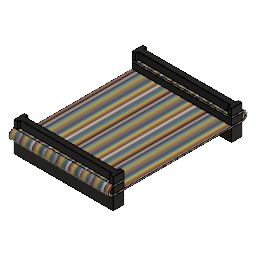
b6c1d7c7-71d5-4f8c-a852-1080e0dc13f3 (Autodesk Fusion 360 design; units mm, degrees)
Autodesk Fusion 360 part; units mm, degrees
note: some values were not read from the file. Set by a fixed rule: which face or edge a step refers to.
sketch "Sketch1" plane through (0, 0, 0) normal (0, 0, 1) x (1, 0, 0) in component "GPIO Header cable v2"
  line L0 (27.75, 3) -> (-27.75, 3)
  line L1 (-27.75, 3) -> (-27.75, -3)
  line L2 (-27.75, -3) -> (27.75, -3)
  line L3 (27.75, -3) -> (27.75, 3)
  line L4 (27.75, 3) -> (-27.75, -3) construction
  line L5 (-27.75, 3) -> (27.75, -3) construction
  line L6 (-1.925, -3) -> (1.925, -3)
  line L7 (1.925, -3) -> (1.925, -3.8)
  line L8 (1.925, -3.8) -> (-1.925, -3.8)
  line L9 (-1.925, -3.8) -> (-1.925, -3)
  dimension "d1" = 55.5
  dimension "d2" = 6
  dimension "d3" = 3.85
  dimension "d4" = 0.8
  constraint perpendicular L0 L1
  constraint parallel L0 L2
  constraint parallel L1 L3
  constraint horizontal L0
  constraint coincident L4 origin
  constraint coincident L5 origin
  constraint horizontal L6
  constraint vertical L7
  constraint horizontal L8
  constraint vertical L9
  constraint midpoint L2 L6
  measures "d1" distance of L1.end L2.end
  measures "d2" distance of L0.end L1.end
  measures "d3" distance of L6.start L6.end
  measures "d4" distance of L6.start L8.end
extrude "Extrude1" add sketch "Sketch1" along normal blind 7 makes body 1 in component "GPIO Header cable v2"
sketch "Sketch2" plane through (0, 0, 7) normal (0, 0, 1) x (-1, 0, 0) in component "GPIO Header cable v2"
  line L0 (-1.925, 3) -> (-27.75, 3)
  line L1 (-27.75, 3) -> (-27.75, -3)
  line L2 (-27.75, -3) -> (27.75, -3)
  line L3 (27.75, -3) -> (27.75, 3)
  line L4 (27.75, 3) -> (1.925, 3)
  line L5 (1.925, 3) -> (1.925, 3.8)
  line L6 (1.925, 3.8) -> (-1.925, 3.8)
  line L7 (-1.925, 3.8) -> (-1.925, 3)
  line L8 (27.75, -3) -> (-27.75, -3)
  line L9 (-27.75, -3) -> (-27.75, 3)
  line L10 (-27.75, 3) -> (27.75, 3)
  line L11 (27.75, 3) -> (27.75, -3)
  constraint horizontal L8
  constraint vertical L9
  constraint horizontal L10
  constraint vertical L11
  constraint coincident L0.end L1.start
  constraint coincident L2.end L3.start
extrude "Extrude2" add sketch "Sketch2" along normal blind 1 separate body contours L0 L1 L2 L3 L4 L8 L9 L10 L11 makes body 2 in component "GPIO Header cable v2"
extrude "Extrude3" add 1 faces at (0.6417, 1, 8) along direction (0, 0, 1) blind 3.5 separate body on bodies 2 makes body 3 in component "GPIO Header cable v2"
extrude "Extrude4" add 1 faces at (0.6417, 1, 11.5) along direction (0, 0, 1) blind 1 separate body on bodies 3 makes body 4 in component "GPIO Header cable v2"
extrude "Extrude5" add 1 faces at (0.6417, 1, 12.5) along direction (0, 0, 1) blind 4 separate body on bodies 4 makes body 5 in component "GPIO Header cable v2"
sketch "Sketch4" plane through (0, 0, 16.5) normal (0, 0, 1) x (-1, 0, 0) in component "GPIO Header cable v2"
  line L0 (27.75, 3) -> (-27.75, 3)
  line L1 (-27.75, 3) -> (-27.75, -3)
  line L2 (-27.75, -3) -> (27.75, -3)
  line L3 (27.75, -3) -> (27.75, 3)
  line L4 (25.625, -3) -> (-25.625, -3)
  line L5 (-25.625, -3) -> (-25.625, -1.5)
  line L6 (-25.625, -1.5) -> (25.625, -1.5)
  line L7 (25.625, -1.5) -> (25.625, -3)
  line L8 (25.625, 1.5) -> (-25.625, 1.5)
  line L9 (-25.625, 1.5) -> (-25.625, 3)
  line L10 (-25.625, 3) -> (25.625, 3)
  line L11 (25.625, 3) -> (25.625, 1.5)
  dimension "d15" = 51.25
  dimension "d16" = 1.5
  dimension "d17" = 1.5
  dimension "d18" = 51.25
  constraint horizontal L4
  constraint vertical L5
  constraint horizontal L6
  constraint vertical L7
  constraint midpoint L2 L4
  constraint horizontal L8
  constraint vertical L9
  constraint horizontal L10
  constraint vertical L11
  constraint midpoint L0 L10
  measures "d15" distance of L4.start L4.end
  measures "d16" distance of L4.start L6.end
  measures "d17" distance of L8.start L10.end
  measures "d18" distance of L8.start L8.end
extrude "Extrude6" cut sketch "Sketch4" against normal blind 4 contours L0 L8 L9 L10 L11 | L2 L4 L5 L6 L7 bodies 5 in component "GPIO Header cable v2"
extrude "Extrude7" add 3 faces at (0.6417, -3, 7.3333) (-19.1417, -3, 7.3333) (10.5333, -3, 7.3333) along direction (0, -1, 0) blind 15 on bodies 2 bodies 2 in component "GPIO Header cable v2"
sketch "Sketch5" plane through (27.75, 0, 0) normal (1, 0, 0) x (0, 1, 0) in component "GPIO Header cable v2"
  line L0 (-3, 8) -> (3, 8)
  line L1 (3, 8) -> (3, 11.5)
  line L2 (3, 11.5) -> (-3, 11.5)
  line L3 (-3, 11.5) -> (-3, 8)
  arc A0 (3, 8) -> (3, 11.5) centre (3, 9.75) ccw
  arc A1 (3, 7) -> (3, 12.5) centre (3, 9.75) ccw
  line L4 (3, 12.5) -> (3, 11.5)
  line L5 (3, 8) -> (3, 7)
  dimension "d23" = 1
  constraint coincident L0.end L1.start
  constraint coincident L1.end L2.start
  constraint tangent L2 A0
  constraint perpendicular L2 L4
  constraint perpendicular L0 L5
extrude "Extrude8" add sketch "Sketch5" against normal blind 55.5 contours A0 A1 L4 L5 bodies 2 4 in component "GPIO Header cable v2"
extrude "Extrude9" add 1 faces at (9.25, -18, 7.3333) along direction (0, -1, 0) blind 15 on bodies 2 bodies 2 in component "GPIO Header cable v2"
sketch "Sketch1 (2)" plane through (0, 0, 0) normal (0, 0, 1) x (1, 0, 0) in component "GPIO Header cable v2 (1)"
  line L0 (27.75, 3) -> (-27.75, 3)
  line L1 (-27.75, 3) -> (-27.75, -3)
  line L2 (-27.75, -3) -> (27.75, -3)
  line L3 (27.75, -3) -> (27.75, 3)
  line L4 (27.75, 3) -> (-27.75, -3) construction
  line L5 (-27.75, 3) -> (27.75, -3) construction
  line L6 (-1.925, -3) -> (1.925, -3)
  line L7 (1.925, -3) -> (1.925, -3.8)
  line L8 (1.925, -3.8) -> (-1.925, -3.8)
  line L9 (-1.925, -3.8) -> (-1.925, -3)
  dimension "d1_1" = 55.5
  dimension "d2_1" = 6
  dimension "d3_1" = 3.85
  dimension "d4_1" = 0.8
  constraint perpendicular L0 L1
  constraint parallel L0 L2
  constraint parallel L1 L3
  constraint horizontal L0
  constraint coincident L4 origin
  constraint coincident L5 origin
  constraint horizontal L6
  constraint vertical L7
  constraint horizontal L8
  constraint vertical L9
  constraint midpoint L2 L6
  measures "d1_1" distance of L1.end L2.end
  measures "d2_1" distance of L0.end L1.end
  measures "d3_1" distance of L6.start L6.end
  measures "d4_1" distance of L6.start L8.end
extrude "Extrude1'" add sketch "Sketch1 (2)" along normal blind 7 separate body makes body 6 in component "GPIO Header cable v2 (1)"
sketch "Sketch2 (2)" plane through (0, 0, 7) normal (0, 0, 1) x (-1, 0, 0) in component "GPIO Header cable v2 (1)"
  line L0 (-1.925, 3) -> (-27.75, 3)
  line L1 (-27.75, 3) -> (-27.75, -3)
  line L2 (-27.75, -3) -> (27.75, -3)
  line L3 (27.75, -3) -> (27.75, 3)
  line L4 (27.75, 3) -> (1.925, 3)
  line L5 (1.925, 3) -> (1.925, 3.8)
  line L6 (1.925, 3.8) -> (-1.925, 3.8)
  line L7 (-1.925, 3.8) -> (-1.925, 3)
  line L8 (27.75, -3) -> (-27.75, -3)
  line L9 (-27.75, -3) -> (-27.75, 3)
  line L10 (-27.75, 3) -> (27.75, 3)
  line L11 (27.75, 3) -> (27.75, -3)
  constraint horizontal L8
  constraint vertical L9
  constraint horizontal L10
  constraint vertical L11
  constraint coincident L0.end L1.start
  constraint coincident L2.end L3.start
extrude "Extrude2'" add sketch "Sketch2 (2)" along normal blind 1 separate body contours L0 L1 L2 L3 L4 L8 L9 L10 L11 makes body 7 in component "GPIO Header cable v2 (1)"
extrude "Extrude3'" add 1 faces at (0.6417, 1, 8) along direction (0, 0, 1) blind 3.5 separate body on bodies 7 makes body 8 in component "GPIO Header cable v2 (1)"
extrude "Extrude4'" add 1 faces at (0.6417, 1, 11.5) along direction (0, 0, 1) blind 1 separate body on bodies 8 makes body 9 in component "GPIO Header cable v2 (1)"
extrude "Extrude5'" add 1 faces at (0.6417, 1, 12.5) along direction (0, 0, 1) blind 4 separate body on bodies 9 makes body 10 in component "GPIO Header cable v2 (1)"
sketch "Sketch4 (2)" plane through (0, 0, 16.5) normal (0, 0, 1) x (-1, 0, 0) in component "GPIO Header cable v2 (1)"
  line L0 (27.75, 3) -> (-27.75, 3)
  line L1 (-27.75, 3) -> (-27.75, -3)
  line L2 (-27.75, -3) -> (27.75, -3)
  line L3 (27.75, -3) -> (27.75, 3)
  line L4 (25.625, -3) -> (-25.625, -3)
  line L5 (-25.625, -3) -> (-25.625, -1.5)
  line L6 (-25.625, -1.5) -> (25.625, -1.5)
  line L7 (25.625, -1.5) -> (25.625, -3)
  line L8 (25.625, 1.5) -> (-25.625, 1.5)
  line L9 (-25.625, 1.5) -> (-25.625, 3)
  line L10 (-25.625, 3) -> (25.625, 3)
  line L11 (25.625, 3) -> (25.625, 1.5)
  dimension "d15_1" = 51.25
  dimension "d16_1" = 1.5
  dimension "d17_1" = 1.5
  dimension "d18_1" = 51.25
  constraint horizontal L4
  constraint vertical L5
  constraint horizontal L6
  constraint vertical L7
  constraint midpoint L2 L4
  constraint horizontal L8
  constraint vertical L9
  constraint horizontal L10
  constraint vertical L11
  constraint midpoint L0 L10
  measures "d15_1" distance of L4.start L4.end
  measures "d16_1" distance of L4.start L6.end
  measures "d17_1" distance of L8.start L10.end
  measures "d18_1" distance of L8.start L8.end
extrude "Extrude6'" cut sketch "Sketch4 (2)" against normal blind 4 contours L0 L8 L9 L10 L11 | L2 L4 L5 L6 L7 bodies 10 in component "GPIO Header cable v2 (1)"
extrude "Extrude7'" add 3 faces at (0.6417, -3, 7.3333) (-19.1417, -3, 7.3333) (10.5333, -3, 7.3333) along direction (0, -1, 0) blind 15 on bodies 7 bodies 7 in component "GPIO Header cable v2 (1)"
sketch "Sketch5 (2)" plane through (27.75, 0, 0) normal (1, 0, 0) x (0, 1, 0) in component "GPIO Header cable v2 (1)"
  line L0 (-3, 8) -> (3, 8)
  line L1 (3, 8) -> (3, 11.5)
  line L2 (3, 11.5) -> (-3, 11.5)
  line L3 (-3, 11.5) -> (-3, 8)
  arc A0 (3, 8) -> (3, 11.5) centre (3, 9.75) ccw
  arc A1 (3, 7) -> (3, 12.5) centre (3, 9.75) ccw
  line L4 (3, 12.5) -> (3, 11.5)
  line L5 (3, 8) -> (3, 7)
  dimension "d23_1" = 1
  constraint coincident L0.end L1.start
  constraint coincident L1.end L2.start
  constraint tangent L2 A0
  constraint perpendicular L2 L4
  constraint perpendicular L0 L5
extrude "Extrude8'" add sketch "Sketch5 (2)" against normal blind 55.5 contours A0 A1 L4 L5 bodies 7 9 in component "GPIO Header cable v2 (1)"
extrude "Extrude9'" add 1 faces at (9.25, -18, 7.3333) along direction (0, -1, 0) blind 15 on bodies 7 bodies 7 in component "GPIO Header cable v2 (1)"
combine "Combine1" operation add target body 2 tool bodies 7 body 7 seen with x (-1, 0, 0) y (0, -1, 0) z (0, 0, 1) at (0, -66, 0) in component "GPIO Header cable v2"
component "GPIO Header cable v2" placed x (1, 0, 0) y (0, 1, 0) z (0, 0, 1) at (0, 0, 0)
component "GPIO Header cable v2 (1)" placed x (-1, 0, 0) y (0, -1, 0) z (0, 0, 1) at (0, -66, 0)
